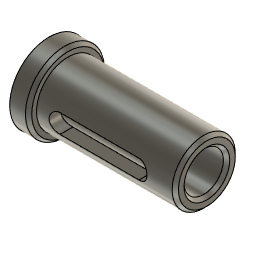
NCV-13 v2 (Autodesk Fusion 360 design; units mm, degrees)
Autodesk Fusion 360 part; units mm, degrees
sketch "Sketch1" plane through (0, 0, 0) normal (0, 1, 0) x (1, 0, 0)
  line L0 (-100, 12.5) -> (-2, 12.5)
  line L1 (-2, 12.5) -> (0, 14.5)
  line L2 (0, 14.5) -> (0, 18)
  line L3 (0, 18) -> (-2, 20)
  line L4 (-2, 20) -> (-88, 20)
  line L5 (-88, 20) -> (-88, 23)
  line L6 (-88, 23) -> (-90, 25)
  line L7 (-90, 25) -> (-100, 25)
  line L8 (-100, 25) -> (-100, 12.5)
  line L9 (0, 0) -> (-74, 0) construction
  line L10 (-74, -6) -> (-24, -6)
  line L11 (-74, 6) -> (-24, 6)
  arc A0 (-74, 6) -> (-74, -6) centre (-74, 0) ccw
  arc A1 (-24, -6) -> (-24, 6) centre (-24, 0) ccw
  dimension "d1" = 88
  dimension "d2" = 100
  dimension "d3" = 135
  dimension "d4" = 25
  dimension "d5" = 20
  dimension "d6" = 100
  dimension "d7" = 14.5
  dimension "d8" = 135
  dimension "d9" = 45
  dimension "d10" = 2
  dimension "d11" = 2
  dimension "d12" = 90
  dimension "d13" = 12
  dimension "d15" = 12
  dimension "d16" = 24
  dimension "d17" = 74
  constraint vertical L2
  constraint vertical L8
  constraint horizontal L7
  constraint vertical L5
  constraint horizontal L4
  constraint horizontal L0
  constraint coincident L9.start origin
  constraint coincident L9.end A0.centre
  constraint horizontal L9
  constraint coincident L9 A1.centre
  constraint horizontal L10
  constraint horizontal L11
  constraint tangent L10 A0
  constraint tangent L11 A0
  measures "d1" horizontal distance of L9.start L4.end
  measures "d2" horizontal distance of L9.start L0.start
  measures "d3" angle of L6 L7
  measures "d4" vertical distance of L9.start L7.end
  measures "d5" vertical distance of L9.start L3.end
  measures "d6" distance of L0.start L2
  measures "d7" distance of L9.start L1.end
  measures "d8" angle of L3 L4
  measures "d9" angle of L1 L2
  measures "d10" horizontal distance of L9.start L3.end
  measures "d11" horizontal distance of L9.start L0.end
  measures "d12" horizontal distance of L9.start L6.end
  measures "d13" diameter of A0
  measures "d15" diameter of A1
  measures "d16" distance of L9.start A1.centre
  measures "d17" distance of L9.start L9.end
revolve "Revolve1" add sketch "Sketch1" angle 360 about axis through (1.75, 0, 0) along (1, 0, 0) contours L0 L1 L2 L3 L4 L5 L6 L7 L8
extrude "Extrude1" cut sketch "Sketch1" against normal through all contours L10 L11 A0 A1
equation "d3 = 180 deg - 45 deg"
equation "d4 = ( 50 / 2 ) * 1 mm"
equation "d5 = ( 40 / 2 ) * 1 mm"
equation "d6 = d2"
equation "d7 = ( 29 / 2 ) * 1 mm"
equation "d12 = d1 + 2 mm"
equation "d17 = d16 + 50 mm"
